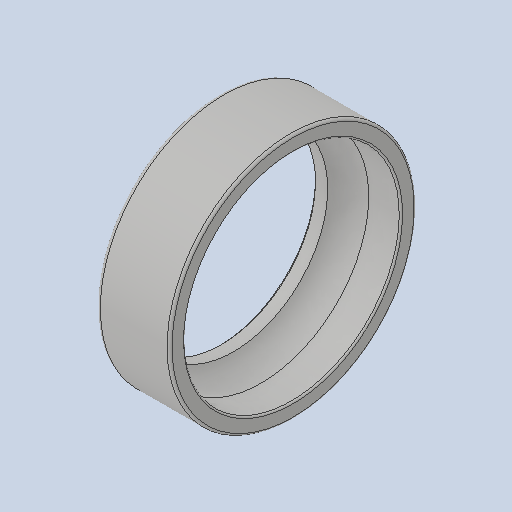
# Autodesk Inventor part: SKF_7200 BECBP_PART2
Saved by Autodesk Inventor 2022 (Build 260153000, 153)
## iProperties
Created: 2022-07-15
Part Number: SKF_7200 BECBP_PART2
Material: Generic
Catalog Web Link: www.cadenas.de
Description: -Angular contact ball bearings, single row
Vendor: SKF
Document SubType Name: Modeling
Designer: psAdmin
Manufacturer: SKF
Mass: 30 g
Surface Area: 20.2384 cm^2
Volume: 1.82269 cm^3
Density: 1 g/cm^3
Appearance: PSOLRGB-175-175-175
Category: PARTsolutions
Company: SKF
PSOL_IDENT_0: {$CADENAS_DATA/23d-libs/skf/bearings_units_and_housings/ball_bearings/angular_contact_ball_bearings/
PSOL_IDENT_1: ba1_001_101.prj},208 {VTYP=3D},{NB=SKF_7200 BECBP_PART2},{LINA=SKF_7200 BECBP_PART2},{NN=BA1_001_101
PSOL_IDENT_2: _PART2},{NOPRJ=TRUE},{DATE=08.07.2022 10:24:26},{GEOMDATE=04.07.2022 06:53:14},{VERSION=},{LINEID=14
PSOL_IDENT_3: 1430},{WBVAR=},{WBNUMERIC=}  {NB=SKF_7200 BECBP_PART2},{LINA=SKF_7200 BECBP_PART2},{KT=DUMMY},{DESIG
PSOL_IDENT_4: NATION=7200 BECBP},{DD=10.000},{D=30.000},{B=9.0000},{DD1=18.300},{DD2=14.570},{D1=22.850},{D2=26.18
PSOL_IDENT_5: 0},{D3=0.000},{D4=26.180},{D5=},{C1=0.000},{AA=13},{R12=0.600},{R34=0.300},{ALPHA=40},{PITCH=20.300}
PSOL_IDENT_6: ,{DW=6.000},{DDAMIN=14.2},{DDAMAX=},{DAMAX=25.8},{DBMAX=27.6},{RAMAX=0.6},{RBMAX=0.3},{LOAD1=7.02},{
PSOL_IDENT_7: LOAD2=3.35},{LOAD3=0.14},{SPEED1=30000},{SPEED2=30000},{Z=9},{II=1},{MASS=0.03},{BEARING=7200 BECBP}
PSOL_IDENT_8: ,{POPULAR=Yes},{VARIANT=acbb1},{D2A=},{DD2A=14.570},{R5R=0.3},{R34L=0.6},{IRH=1},{ORH=1},{D4H=0.6}
NB: SKF_7200 BECBP_PART2
NT: Angular contact ball bearings, single row
NBSYN: SKF_$DESIGNATION._PART2
LINA: SKF_7200 BECBP_PART2
CATALOG: SKF
DESIGNATION: 7200 BECBP
DD: 10
D: 30
B: 9
LOAD1: 7.02
LOAD2: 3.35
LOAD3: 0.14
SPEED1: 30000
SPEED2: 30000
SUPPLIER: SKF
ARTICLENO: SKF_7200 BECBP_PART2
BOMINFO: SKF_7200 BECBP_PART2
CREATOR: CADENAS GmbH
Title: SKF_7200 BECBP_PART2
Author: Cadenas PARTsolutions
Comments: Angular contact ball bearings, single row
Autodesk Inventor part; units mm, degrees
ref_plane "YZ Plane" through (0, 0, 0) normal (1, 0, 0) x (0, 1, 0)
ref_plane "XZ Plane" through (0, 0, 0) normal (0, 1, 0) x (-1, 0, 0)
ref_plane "XY Plane" through (0, 0, 0) normal (0, 0, 1) x (1, 0, 0)
sketch "Sketch_1" plane through (0, 0, 0) normal (0, 0, 1) x (1, 0, 0)
  line L0 (9, 0) -> (0, 0)
  line L1 (0, 11.725) -> (0.3, 11.425)
  line L2 (0.3, 11.425) -> (1.7844, 11.425)
  arc A0 (5.097, 13.09) -> (1.7844, 11.425) centre (4.5, 10.15) ccw
  line L3 (5.097, 13.09) -> (8.8, 13.09)
  arc A1 (8.8, 13.09) -> (9, 13.29) centre (8.8, 13.29) ccw
  line L4 (9, 13.29) -> (9, 14.7)
  arc A2 (9, 14.7) -> (8.7, 15) centre (8.7, 14.7) ccw
  line L5 (8.7, 15) -> (0.6, 15)
  arc A3 (0.6, 15) -> (0, 14.4) centre (0.6, 14.4) ccw
  line L6 (0, 14.4) -> (0, 11.725)
  constraints: 14 end point, 8 point on circle, 4 centre point
revolve "Revolution1" add sketch "Sketch_1" angle 360 about axis through (9, 0, 0) along (1, 0, 0)
body "Solid1"
